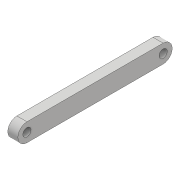
# Autodesk Inventor part: Link_Principal
Saved by Autodesk Inventor 2018 (Build 220112000, 112)
## iProperties
Created: 2021-04-28
Part Number: Link_Principal
Material: Generic
Document SubType Name: Modeling
Designer: l01767
Density: 1 g/cm^3
Appearance: Default
Author: l01767
Autodesk Inventor part; units mm, degrees
ref_plane "YZ Plane" through (0, 0, 0) normal (1, 0, 0) x (0, 1, 0)
ref_plane "XZ Plane" through (0, 0, 0) normal (0, 1, 0) x (-1, 0, 0)
ref_plane "XY Plane" through (0, 0, 0) normal (0, 0, 1) x (1, 0, 0)
sketch "Sketch1" plane through (0, 0, 0) normal (1, 0, 0) x (0, 1, 0)
  line L0 (-300, 0) -> (300, 0) construction
  line L1 (-300, -40) -> (300, -40)
  line L2 (300, 40) -> (-300, 40)
  arc A0 (-300, 40) -> (-300, -40) centre (-300, 0) ccw
  arc A1 (300, -40) -> (300, 40) centre (300, 0) ccw
  circle A2 centre (300, 0) radius 18
  line L3 (0, 0) -> (0, -40)
  circle A3 centre (-300, 0) radius 18
  dimension "d0" = 300
  dimension "d1" = 80
  dimension "d2" = 36
  constraints: 10 end point, 4 centre point, 4 point on circle, 4 tangent, 2 midpoint, 1 coincident, 1 horizontal, 1 parallel, 1 symmetric about line, 1 other
  measures "d0" distance of L3.start L0.end
  measures "d1" distance between parallel lines of L2 L1
  measures "d2" diameter of A2
extrude "Extrusion1" add sketch "Sketch1" along normal mid plane 44.45
body "Solid1"
